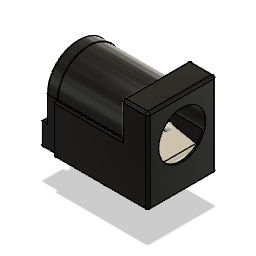
Power_Jack (Autodesk Fusion 360 design; units mm, degrees)
Autodesk Fusion 360 part; units mm, degrees
note: some values were not read from the file. Set by a fixed rule: which sketch regions a step uses.
sketch "Sketch1" plane through (0, 0, 0) normal (0, 0, 1) x (1, 0, 0)
  line L0 (-4.38, 10.8) -> (4.38, 10.8)
  line L1 (4.38, 10.8) -> (4.38, 0)
  line L2 (4.38, 0) -> (-4.38, 0)
  line L3 (-4.38, 0) -> (-4.38, 10.8)
  dimension "d1" = 8.76
  dimension "d2" = 10.8
  dimension "d3" = 4.38
  constraint horizontal L0
  constraint vertical L1
  constraint horizontal L2
  constraint vertical L3
  constraint coincident origin L2
  measures "d1" distance of L0.start L0.end
  measures "d2" distance of L0.start L2.end
  measures "d3" distance of origin L3
extrude "Extrude1" add sketch "Sketch1" against normal blind 13.34
ref_plane "WorkPlane1" through (0, 5.4, -3.4) normal (0, 0, 1) x (1, 0, 0)
sketch "Sketch2" plane through (0, 5.4, -3.4) normal (0, 0, 1) x (1, 0, 0)
  line L0 (-3.98, -5.4) -> (-3.98, 0.84)
  arc A0 (3.98, 0.84) -> (-3.98, 0.84) centre (0, 0.84) ccw
  line L1 (3.98, 0.84) -> (3.98, -5.4)
  line L2 (4.38, -5.4) -> (-4.38, -5.4)
  line L3 (-3.98, 0.84) -> (-4.38, 0.84)
  line L4 (-4.38, -5.4) -> (-4.38, 5.4)
  line L5 (0, 0) -> (0, -2)
  line L6 (3.98, 0.84) -> (4.38, 0.84)
  line L7 (-4.38, 0.84) -> (-4.38, 5.4)
  line L8 (-4.38, 5.4) -> (4.38, 5.4)
  line L9 (4.38, 5.4) -> (4.38, 0.84)
  line L10 (-4.03, -5.4) -> (-4.03, 0.84)
  arc A1 (4.03, 0.84) -> (-4.03, 0.84) centre (0, 0.84) ccw
  line L11 (4.03, 0.84) -> (4.03, -5.4)
  line L12 (4.38, 0.84) -> (4.38, -5.4)
  point P0 (0, 4.82)
  point P1 (4.38, 5.4)
  dimension "d7" = 10.22
  dimension "d8" = 7.96
  dimension "d12" = 0.05
  constraint vertical L0
  constraint tangent L0 A0
  constraint tangent A0 L1
  constraint parallel L0 L1
  constraint vertical L5.start A0.centre
  constraint midpoint A0 P0
  constraint coincident L0 A0.end
  constraint perpendicular L0 L3
  constraint coincident L3.end L4
  constraint coincident L5.start origin
  constraint vertical L5
  constraint symmetric L0.end L5 A0.start
  constraint symmetric L3.end L5 L6.end
  constraint coincident L4.end L7.end
  constraint coincident P1 L8.end
  constraint coincident L0.end L3
  constraint coincident L1.end L2
  constraint coincident L0.start L2
  constraint coincident L2.start L12.end
  measures "d7" distance of P0 L2
  measures "d8" distance of L0 L1
extrude "Extrude2" cut sketch "Sketch2" against normal blind 9.94 contours A0 L3 L6 A1 | L3 L4 L6 L7 L8 L9 A1
extrude "Extrude3" add sketch "Sketch2" along normal blind 1.44 from surface at -9.94 contours A0 L3 L6 A1
extrude "Extrude4" cut sketch "Sketch2" along normal blind 1.44 from surface at -9.94 contours L2 L3 L4 L10 | L2 L6 L11 L12
sketch "Sketch3" plane through (0, 0, 0) normal (0, 0, 1) x (1, 0, 0)
  line L0 (-4.38, 0) -> (4.38, 0)
  line L1 (4.38, 0) -> (4.38, 10.8)
  line L2 (4.38, 10.8) -> (-4.38, 10.8)
  line L3 (-4.38, 10.8) -> (-4.38, 0)
  circle A0 centre (0, 6.32) radius 3
  point P0 (0, 3.32)
  dimension "d19" = 6
  dimension "d20" = 3.32
  constraint coincident A0 P0
  constraint vertical A0.centre P0
  constraint vertical origin A0.centre
  measures "d19" diameter of A0
  measures "d20" distance of origin P0
extrude "Extrude5" cut sketch "Sketch3" against normal blind 10 contours A0
ref_plane "WorkPlane2" through (0, 5.4, -0.2) normal (0, 0, 1) x (1, 0, 0)
sketch "Sketch4" plane through (0, 5.4, -0.2) normal (0, 0, 1) x (1, 0, 0)
  line L0 (-2.98, -0.0107) -> (2.98, -0.0107)
  line L1 (2.98, -0.0107) -> (2.98, -4.4)
  line L2 (2.98, -4.4) -> (-2.98, -4.4)
  line L3 (-2.98, -4.4) -> (-2.98, -0.0107)
  line L4 (4.38, -5.4) -> (4.38, 0.84)
  line L5 (-4.38, 0.84) -> (-4.38, -5.4)
  line L6 (4.03, -5.4) -> (-4.03, -5.4)
  dimension "d24" = 1.4
  dimension "d25" = 1.4
  dimension "d26" = 1
  constraint horizontal L0
  constraint vertical L1
  constraint horizontal L2
  constraint vertical L3
  measures "d24" distance of L1 L4
  measures "d25" distance of L3 L5
  measures "d26" distance of L2 L6
extrude "Extrude6" cut sketch "Sketch4" against normal blind 9.8
sketch "Sketch5" plane through (0, 0, -10) normal (0, 0, 1) x (1, 0, 0)
  arc A0 (2.852, 5.3893) -> (-2.852, 5.3893) centre (0, 6.32) ccw
  line L0 (-2.852, 5.3893) -> (-2.98, 5.3893)
  line L1 (-2.98, 5.3893) -> (-2.98, 1)
  line L2 (-2.98, 1) -> (2.98, 1)
  line L3 (2.98, 1) -> (2.98, 5.3893)
  line L4 (2.98, 5.3893) -> (2.852, 5.3893)
  circle A1 centre (0, 6.32) radius 3
  circle A2 centre (0, 6.32) radius 0.5
  circle A3 centre (0, 6.32) radius 0.75
  dimension "d29" = 1
  dimension "d30" = 1.5
  constraint concentric A1 A2
  constraint concentric A1 A3
  measures "d29" diameter of A2
  measures "d30" diameter of A3
extrude "Extrude7" add sketch "Sketch5" along normal blind 8.6 contours A2
extrude "Extrude8" add sketch "Sketch5" along normal blind 0.3 contours A3
fillet "Fillet1" radius 0.5 1 edges at (-0.4662, 6.1392, -1.4)
extrude "Extrude9" add sketch "Sketch5" against normal blind 3.74 contours A3
extrude "Extrude10" cut 1 faces at (0.3052, 6.1649, -13.34) along direction (0, 0, 1) blind 0.1
fillet "Fillet2" radius 0.5 1 edges at (-0.4662, 6.1392, -13.24)
sketch "Sketch6" plane through (0, 0, -13.34) normal (0, 0, -1) x (-1, 0, 0)
  line L0 (-4.03, 6.24) -> (-4.03, 0)
  line L1 (-4.03, 0) -> (4.03, 0)
  line L2 (4.03, 0) -> (4.03, 6.24)
  arc A0 (4.03, 6.24) -> (-4.03, 6.24) centre (0, 6.24) ccw
  circle A1 centre (0, 6.32) radius 0.75
  circle A2 centre (0, 6.32) radius 0.5
  circle A3 centre (0, 6.32) radius 0.75
  line L3 (-1.55, 4.9784) -> (-1.55, 2.9784)
  line L4 (0, 0) -> (0, -4.4876) construction
  line L5 (-1.55, 2.9784) -> (-0.8135, -3.0203)
  arc A4 (-0.8135, -3.0203) -> (0.8135, -3.0203) centre (0, -2.9204) ccw
  line L6 (1.55, 4.9784) -> (1.55, 2.9784)
  line L7 (1.55, 2.9784) -> (0.8135, -3.0203)
  arc A5 (1.55, 4.9784) -> (-1.55, 4.9784) centre (0, 6.32) ccw
  circle A6 centre (0, -2.9204) radius 0.35
  line L8 (-1.55, 2.9784) -> (-4.03, 2.9784)
  line L9 (-4.03, 2.9784) -> (-4.03, 0)
  line L10 (-4.03, 0) -> (-1.1843, 0)
  line L11 (1.55, 2.9784) -> (4.03, 2.9784)
  line L12 (4.03, 2.9784) -> (4.03, 0)
  line L13 (4.03, 0) -> (1.1843, 0)
  point P0 (0, -3.74)
  dimension "d41" = 4.1
  dimension "d42" = 1.55
  dimension "d43" = 2
  dimension "d46" = 173
  dimension "d47" = 3.74
  dimension "d48" = 0.7
  constraint concentric A2 A5
  constraint vertical L3
  constraint coincident L4.start origin
  constraint perpendicular L1 L4
  constraint tangent L5 A4
  constraint vertical L4.start A4.centre
  constraint midpoint A4 P0
  constraint symmetric L3.start L4 L6.start
  constraint symmetric L3.end L4 L6.end
  constraint symmetric L4 L5.end A4.end
  constraint concentric A4 A6
  constraint horizontal L8
  constraint vertical L9
  constraint horizontal L10
  constraint coincident L0.end L1.start
  constraint horizontal L11
  constraint vertical L12
  constraint horizontal L13
  constraint coincident L1.end L2.start
  constraint coincident L5 L10.end
  constraint coincident L7 L13.end
  measures "d41" diameter of A5
  measures "d42" distance of L4.start L3
  measures "d43" distance of L3.start L3.end
  measures "d46" angle of L3 L5
  measures "d47" distance of L1 P0
  measures "d48" diameter of A6
extrude "Extrude11" add sketch "Sketch6" along normal blind 0.2 contours L1 L3 L5 L6 L7 A5 | L1 L5 A4 L7
extrude "Extrude12" add sketch "Sketch6" along normal blind 0.7 contours L0 L1 L5 L8 L9 L10 | L1 L2 L7 L11 L12 L13
sketch "Sketch7" plane through (0, 0, -11.9) normal (0, 0, -1) x (-1, 0, 0)
  line L0 (-4.03, 0) -> (-4.03, 6.24)
  line L1 (-4.03, 6.24) -> (-4.38, 6.24)
  line L2 (-4.38, 6.24) -> (-4.38, 0)
  line L3 (-4.38, 0) -> (-4.03, 0)
  line L4 (-3.3138, 4) -> (-4.4, 4)
  line L5 (-4.6, 3.8) -> (-4.6, -4.261)
  line L6 (-3.3138, 3.8) -> (-4.2, 3.8)
  line L7 (-4.4, 3.6) -> (-4.4, -4.261)
  line L8 (-3.3138, 4) -> (-3.3138, 3.8)
  line L9 (-4.6, -4.261) -> (-4.4, -4.261)
  arc A0 (-4.2, 3.8) -> (-4.4, 3.6) centre (-4.2, 3.6) ccw
  arc A1 (-4.4, 4) -> (-4.6, 3.8) centre (-4.4, 3.8) ccw
  dimension "d54" = 0.02
  dimension "d55" = 4
  dimension "d58" = 0.2
  constraint perpendicular L0 L4
  constraint perpendicular L4 L5
  constraint parallel L4 L6
  constraint parallel L5 L7
  constraint tangent L6 A0
  constraint tangent L7 A0
  constraint tangent L4 A1
  constraint tangent L5 A1
  constraint equal A0 A1
  measures "d54" distance of L2.end L7
  measures "d55" distance of L2.end L4
  measures "d58" radius of A0
extrude "Extrude13" add sketch "Sketch7" against normal blind 2.44 contours L2 L4 L5 L7 L9 A0 A1
sketch "Sketch8" plane through (4.6, 0, 0) normal (1, 0, 0) x (0, 0, -1)
  line L0 (11.9, -4.261) -> (11.9, 3.8)
  line L1 (11.9, 3.8) -> (9.46, 3.8)
  line L2 (9.46, 3.8) -> (9.46, -4.261)
  line L3 (9.46, -4.261) -> (11.9, -4.261)
  arc A0 (9.46, -2.56) -> (11.9, -2.56) centre (10.68, -2.56) ccw
  line L4 (0, 0) -> (11.9, 0)
  circle A1 centre (10.68, -2.56) radius 0.35
  point P0 (10.68, -3.78)
  dimension "d59" = 3.78
  dimension "d60" = 0.7
  constraint coincident L2 A0.start
  constraint horizontal A0.start A0.end
  constraint coincident L0 A0.end
  constraint midpoint A0 P0
  constraint tangent L2 A0
  constraint concentric A0 A1
  measures "d59" distance of P0 L4
  measures "d60" diameter of A1
extrude "Extrude14" cut sketch "Sketch8" against normal blind 2.2 contours L0 L2 L3 A0 | A1
sketch "Sketch9" plane through (0, 0, 0) normal (0, -1, 0) x (1, 0, 0)
  line L0 (4.03, -14.04) -> (4.03, -11.9)
  line L1 (4.03, -11.9) -> (4.38, -11.9)
  line L2 (4.38, -11.9) -> (4.38, 0)
  line L3 (4.38, 0) -> (-4.38, 0)
  line L4 (-4.38, 0) -> (-4.38, -11.9)
  line L5 (-4.38, -11.9) -> (-4.03, -11.9)
  line L6 (-4.03, -11.9) -> (-4.03, -14.04)
  line L7 (-4.03, -14.04) -> (-1.1843, -14.04)
  line L8 (-1.1843, -14.04) -> (-1.1843, -13.54)
  line L9 (-1.1843, -13.54) -> (-1.1843, -13.34)
  line L10 (-1.1843, -13.34) -> (1.1843, -13.34)
  line L11 (1.1843, -13.34) -> (1.1843, -13.54)
  line L12 (1.1843, -13.54) -> (1.1843, -14.04)
  line L13 (1.1843, -14.04) -> (4.03, -14.04)
  line L14 (-1.1, -9.14) -> (1.1, -9.14)
  line L15 (1.1, -9.14) -> (1.1, -8.94)
  line L16 (1.1, -8.94) -> (-1.1, -8.94)
  line L17 (-1.1, -8.94) -> (-1.1, -9.14)
  dimension "d63" = 4.2
  dimension "d64" = 0.2
  dimension "d65" = 2.2
  dimension "d66" = 1.1
  constraint horizontal L14
  constraint vertical L15
  constraint horizontal L16
  constraint vertical L17
  measures "d63" distance of L10 L14
  measures "d64" distance of L14 L16
  measures "d65" distance of L15.end L16.end
  measures "d66" horizontal distance of origin L16.end
extrude "Extrude15" add sketch "Sketch9" along normal blind 6.5 contours L14 L15 L16 L17
sketch "Sketch10" plane through (0, 0, -8.94) normal (0, 0, 1) x (1, 0, 0)
  line L0 (1.1, 0) -> (-1.1, 0)
  line L1 (-1.1, 0) -> (-1.1, -6.5)
  line L2 (-1.1, -6.5) -> (1.1, -6.5)
  line L3 (1.1, -6.5) -> (1.1, 0)
  arc A0 (-1.1, -2.68) -> (1.1, -2.68) centre (0, -2.68) ccw
  line L4 (4.38, 0) -> (-4.38, 0)
  circle A1 centre (0, -2.68) radius 0.35
  point P0 (0, -3.78)
  dimension "d69" = 3.78
  dimension "d70" = 0.7
  constraint horizontal A0.end A0.start
  constraint coincident L3 A0.end
  constraint coincident L1 A0.start
  constraint midpoint A0 P0
  constraint tangent L1 A0
  constraint concentric A0 A1
  measures "d69" distance of P0 L4
  measures "d70" diameter of A1
extrude "Extrude16" cut sketch "Sketch10" against normal blind 0.2 contours L1 L2 L3 A0 | A1
ref_plane "WorkPlane3" through (2.68, 3.1947, -5.1) normal (-1, 0, 0) x (0, 1, 0)
sketch "Sketch11" plane through (2.68, 3.1947, -5.1) normal (-1, 0, 0) x (0, 0, -1)
  arc A0 (4.1199, -2.0972) -> (4.6, -1.7053) centre (4.2, -1.7053) ccw
  line L0 (4.1199, -2.0972) -> (-4.2201, -0.3932)
  arc A1 (-4.548, 0.5938) -> (-4.2201, -0.3932) centre (-4.1, 0.1947) ccw
  line L1 (-4.548, 0.5938) -> (-3.122, 2.1947)
  line L2 (4.6, 2.1947) -> (4.6, -1.7053)
  line L3 (4.9, 2.1947) -> (4.9, -2.1947)
  line L4 (-4.9, 2.1947) -> (4.9, 2.1947)
  line L5 (-5.1, 3.1947) -> (-5.1, -7.6053)
  dimension "d74" = 0.3
  dimension "d75" = 3.9
  dimension "d76" = 2
  dimension "d77" = 0.6
  dimension "d78" = 1
  dimension "d79" = 0.4
  constraint tangent L0 A1
  constraint tangent A1 L1
  constraint vertical L2
  constraint coincident A0.end L2.end
  constraint tangent A0 L0
  constraint tangent A0 L2
  constraint coincident L1.end L4
  constraint coincident L2.start L4
  measures "d74" distance of L2 L3
  measures "d75" distance of A0.centre L4
  measures "d76" distance of A1.centre L4
  measures "d77" radius of A1
  measures "d78" distance of A1.centre L5
  measures "d79" radius of A0
extrude "Extrude18" add sketch "Sketch11" along normal blind 5.36
fillet "Fillet3" radius 0.3 8 edges at (4.38, 10.8, -1.7) (0, 10.8, 0) (0, 10.8, -3.4) (-4.38, 10.8, -1.7) (4.38, 5.4, 0) (-4.38, 5.4, 0) (4.38, 8.52, -3.4) (-4.38, 8.52, -3.4)
fillet "Fillet4" radius 0.2 20 edges at (4.38, 6.24, -7.5) (-4.38, 0, -6.1) (-4.2921, 0, -0.0879) (0, 0, 0) (4.2921, 0, -0.0879) (4.38, 0, -6.1) (-4.38, 6.24, -7.5) (4.03, 4.6092, -13.34) (0, 10.27, -13.34) (-4.03, 4.6092, -13.34) (-2.79, 2.9784, -14.04) (-1.3672, 1.4892, -14.04) (1.3672, 1.4892, -14.04) (2.79, 2.9784, -14.04) (2.6072, 0, -14.04) (-2.6072, 0, -14.04) (-4.03, 0, -12.97) (4.03, 0, -12.97) (-4.03, 1.4892, -14.04) (4.03, 1.4892, -14.04)
sketch "Sketch12" plane through (0, 0, -11.9) normal (0, 0, -1) x (-1, 0, 0)
  arc A0 (-4.38, 0.2) -> (-4.18, 0) centre (-4.18, 0.2) ccw
  line L0 (-4.18, 0) -> (-3.83, 0)
  arc A1 (-4.03, 0.2) -> (-3.83, 0) centre (-3.83, 0.2) ccw
  line L1 (-4.03, 0.2) -> (-4.03, 6.24)
  line L2 (-4.03, 6.24) -> (-4.18, 6.24)
  arc A2 (-4.18, 6.24) -> (-4.38, 6.04) centre (-4.18, 6.04) ccw
  line L3 (-4.38, 6.04) -> (-4.38, 4)
  line L4 (-4.38, 4) -> (-4.4, 4)
  arc A3 (-4.4, 4) -> (-4.6, 3.8) centre (-4.4, 3.8) ccw
  line L5 (-4.6, 3.8) -> (-4.6, -2.56)
  line L6 (-4.6, -2.56) -> (-4.4, -2.56)
  line L7 (-4.4, -2.56) -> (-4.4, 3.6)
  arc A4 (-4.38, 3.6872) -> (-4.4, 3.6) centre (-4.2, 3.6) ccw
  line L8 (-4.38, 3.6872) -> (-4.38, 0.2)
  line L9 (-4.38, 3.6872) -> (-4.38, 4)
  constraint coincident A4.start L8.start
  constraint coincident L3.end L4.start
split_face "SplitFace1" 1 faces at (4.1467, 3.48, -11.9) by curves path "Sketch12" along L9
move_body "Move1" bodies 1 to x (0, 0, -1) y (0, 1, 0) z (1, 0, 0) at (9.659, 0, -18.421)
equation "d3 = d1 / 2"
equation "d27 = -10 mm + 0.2 mm"
equation "d31 = 10 mm - 1.4 mm"
equation "d36 = -3.54 mm - 0.2 mm"
equation "d42 = ( 3.1 / 2 ) * 1 mm"
equation "d66 = d65 / 2"
equation "d82 = 5.66 mm - 0.3 mm"
